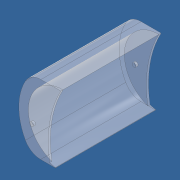
# Autodesk Inventor part: Shovel
Saved by Autodesk Inventor 2021 (Build 250183000, 183)
## iProperties
Created: 2021-03-26
Part Number: Shovel
Material: Generic
Document SubType Name: Modeling
Designer: gurle
Density: 1 g/cm^3
Appearance: Polycarbonate - Clear
Author: gurle
Autodesk Inventor part; units mm, degrees
ref_plane "YZ Plane" through (0, 0, 0) normal (1, 0, 0) x (0, 1, 0)
ref_plane "XZ Plane" through (0, 0, 0) normal (0, 1, 0) x (-1, 0, 0)
ref_plane "XY Plane" through (0, 0, 0) normal (0, 0, 1) x (1, 0, 0)
sketch "Sketch1" plane through (0, 0, 0) normal (0, 0, 1) x (1, 0, 0)
  arc A0 (-163.6506, -118.3654) -> (-93.4502, -160) centre (-93.4502, -80) ccw
  line L0 (-92.0944, 160) -> (0, 160)
  line L1 (0, 160) -> (-92.0944, 160)
  arc A1 (0, 160) -> (-51.3175, -151.5471) centre (426.5438, -70.2596) ccw
  arc A2 (-51.3175, -151.5471) -> (-25.1411, -158.0124) centre (0, 0) ccw
  arc A3 (0, 160) -> (-25.1411, -158.0124) centre (0, 0) ccw
  line L2 (-93.4502, -160) -> (-25.2982, -160)
  arc A4 (-25.2982, -160) -> (-25.1411, -158.0124) centre (-25.2982, -159) ccw
  line L3 (-25.2982, -160) -> (-93.4502, -160)
  arc A5 (-163.6506, -118.3654) -> (-93.4502, -160) centre (-93.4502, -80) ccw
  arc A6 (-163.6414, 118.3822) -> (-163.6506, -118.3654) centre (52.9327, 0) ccw
  arc A7 (-92.0944, 160) -> (-163.6414, 118.3822) centre (-93.444, 80.0114) ccw
  point P0 (-51.3175, -151.5471)
  dimension "d53" = 160
  dimension "d55" = 68.152
  dimension "d56" = 80
  dimension "d60" = 92.0944
  dimension "d65" = 1
  dimension "d66" = 484.7258
  dimension "d71" = 246.8171
  dimension "d72" = 80
  constraints: 16 point on circle, 8 centre point, 8 end point, 2 collinear, 2 tangent, 1 concentric
  measures "d53" radius of A3
  measures "d55" distance of L3.end L3.start
  measures "d56" radius of A0
  measures "d60" distance of L0.end L0.start
  measures "d65" radius of A4
  measures "d66" radius of A1
  measures "d71" radius of A6
  measures "d72" radius of A7
extrude "Extrusion1" add sketch "Sketch1" along normal mid plane 442.6 contours A6 A7 L0 A3 A2 A4 L2 A0
sketch "Sketch2" plane through (0, 0, 221.3) normal (0, 0, 1) x (1, 0, 0)
  arc A0 (-51.3175, -151.5471) -> (-25.1411, -158.0124) centre (0, 0) ccw
  line L0 (-25.2982, -160) -> (-93.4502, -160)
  arc A1 (-25.2982, -160) -> (-25.1411, -158.0124) centre (-25.2982, -159) ccw
  line L1 (-93.4502, -160) -> (-25.2982, -160)
  arc A2 (-163.6506, -118.3654) -> (-93.4502, -160) centre (-93.4502, -80) ccw
  arc A3 (-163.6506, -118.3654) -> (-93.4502, -160) centre (-93.4502, -80) ccw
  line L2 (-92.0944, 160) -> (0, 160)
  line L3 (0, 160) -> (-92.0944, 160)
  arc A4 (0, 160) -> (-51.3175, -151.5471) centre (426.5438, -70.2596) ccw
  arc A5 (0, 160) -> (-25.1411, -158.0124) centre (0, 0) ccw
  arc A6 (-163.6414, 118.3822) -> (-163.6506, -118.3654) centre (52.9327, 0) ccw
  arc A7 (-92.0944, 160) -> (-163.6414, 118.3822) centre (-93.444, 80.0114) ccw
  dimension "d73" = 160
  dimension "d74" = 68.152
  dimension "d75" = 80
  dimension "d76" = 92.0944
  dimension "d77" = 1
  dimension "d78" = 484.7258
  dimension "d79" = 246.8171
  dimension "d80" = 80
  constraints: 16 point on circle, 8 centre point, 8 end point, 2 collinear, 2 tangent, 1 concentric
  measures "d73" radius of A5
  measures "d74" distance of L0.end L0.start
  measures "d75" radius of A2
  measures "d76" distance of L2.end L2.start
  measures "d77" radius of A1
  measures "d78" radius of A4
  measures "d79" radius of A6
  measures "d80" radius of A7
extrude "Extrusion2" add sketch "Sketch2" along normal blind 10
sketch "Sketch10" plane through (0, 0, 231.3) normal (0, 0, 1) x (1, 0, 0)
  circle A0 centre (-125.0944, -30) radius 9
  line L0 (-93.4502, -160) -> (-25.2982, -160) projected
  arc A1 (-25.2982, -160) -> (-25.1411, -158.0124) centre (-25.2982, -159) ccw projected
  point P0 (0, 0)
  dimension "d81" = 18
  dimension "d82" = 130
  dimension "d83" = 99.7962
  constraints: 1 centre point
  measures "d81" diameter of A0
  measures "d82" distance from line of A0.centre L0
  measures "d83" horizontal distance of A1.centre A0.centre
extrude "Extrusion9" add sketch "Sketch10" along normal blind 9.7
mirror "Mirror4" about plane through (0, 0, 0) normal (0, 0, 1) of "Extrusion2", "Extrusion9"
body "Solid1"
